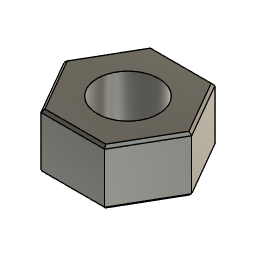
M5 nut v1 (Autodesk Fusion 360 design; units mm, degrees)
Autodesk Fusion 360 part; units mm, degrees
sketch "Sketch1" plane through (0, 0, 0) normal (0, 0, 1) x (1, 0, 0)
  circle A0 centre (0, 0) radius 2.5
  line L0 (0, 0) -> (5, 8.6603) construction
  line L1 (0, 0) -> (5, -8.6603) construction
  line L2 (0, 0) -> (-5, -8.6603) construction
  line L3 (0, 0) -> (-5, 8.6603) construction
  line L4 (10, 0) -> (-10, 0) construction
  line L5 (2.5981, 4.5) -> (5.1962, 0)
  line L6 (5.1962, 0) -> (2.5981, -4.5)
  line L7 (-2.5981, -4.5) -> (-5.1962, 0)
  line L8 (-5.1962, 0) -> (-2.5981, 4.5)
  line L9 (-2.5981, -4.5) -> (2.5981, -4.5)
  line L10 (-2.5981, 4.5) -> (2.5981, 4.5)
  dimension "d1" = 5
  constraint coincident A0.centre L0.start
  constraint coincident L0 L5.start
  constraint coincident L1 L6.end
  constraint coincident L2 L7.start
  constraint coincident L3 L8.end
  constraint coincident L4 L5.end
  constraint coincident L4 L7.end
  constraint parallel L5 L7
  constraint parallel L6 L8
  constraint horizontal L9
  measures "d1" diameter of A0
extrude "Extrude1" add sketch "Sketch1" along normal blind 4.5
chamfer "Chamfer1" distance 0.2 angle 45 12 edges at (0, -4.5, 4.5) (-3.8971, -2.25, 4.5) (-3.8971, 2.25, 4.5) (0, 4.5, 4.5) (3.8971, 2.25, 4.5) (3.8971, -2.25, 4.5) (0, -4.5, 0) (-3.8971, -2.25, 0) (-3.8971, 2.25, 0) (0, 4.5, 0) (3.8971, 2.25, 0) (3.8971, -2.25, 0)
